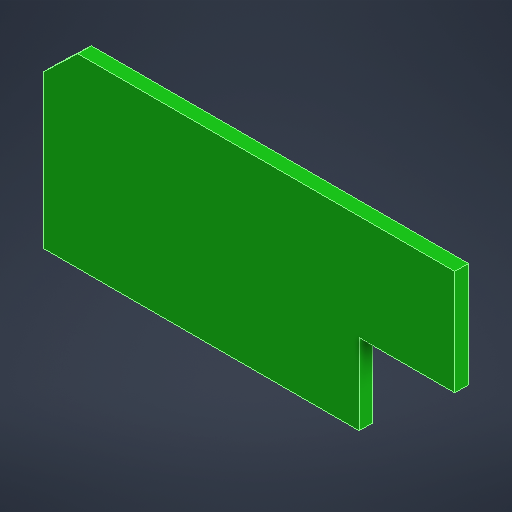
# Autodesk Inventor part: PCB_Dummy
Saved by Autodesk Inventor 2026.2 (Build 302298000, 298)
## iProperties
Created: 2026-01-30
Part Number: PCB_Dummy
Material: PBT plast
Document SubType Name: Modeling
Designer: Vitek
Density: 1.31 g/cm^3
Appearance: Tmavě zelená
Author: Vitek
Autodesk Inventor part; units mm, degrees
ref_plane "YZ Plane" through (0, 0, 0) normal (1, 0, 0) x (0, 1, 0)
ref_plane "XZ Plane" through (0, 0, 0) normal (0, 1, 0) x (-1, 0, 0)
ref_plane "XY Plane" through (0, 0, 0) normal (0, 0, 1) x (1, 0, 0)
sketch "Náčrt1" plane through (0, 0, 0) normal (0, 0, 1) x (1, 0, 0)
  line L0 (-62.75, 34) -> (75.25, 34)
  line L1 (75.25, 34) -> (75.25, -4.5)
  line L2 (40.25, -34) -> (-75.25, -34)
  line L3 (-75.25, -34) -> (-75.25, 22)
  line L4 (-75.25, 22) -> (-62.75, 34)
  line L5 (-112.35, 0) -> (147.35, 0) projected
  line L6 (0, 47.6) -> (0, -47.6) projected
  line L7 (75.25, -4.5) -> (40.25, -4.5)
  line L8 (75.25, -4.5) -> (110.25, -4.5) construction
  line L9 (40.25, -4.5) -> (40.25, -34)
  point P0 (0, 0)
  dimension "d0" = 115.5
  dimension "d4" = 12.5
  dimension "d5" = 12
  dimension "d6" = 35
  dimension "d7" = 180
  dimension "d8" = -29.5
  dimension "d9" = 68
  constraints: 16 end point, 3 parallel, 2 horizontal, 2 perpendicular, 1 collinear, 2 other
  measures "d0" distance of L2.start L2.end
  measures "d4" horizontal distance of L3.end L0.start
  measures "d5" vertical distance of L3.end L0.start
  measures "d6" distance of L1.end L7.end
  measures "d7" angle of L7 L8
  measures "d8" distance between parallel lines of L2 L7
  measures "d9" distance between parallel lines of L2 L0
extrude "Vysunutí1" add sketch "Náčrt1" along normal mid plane 5
